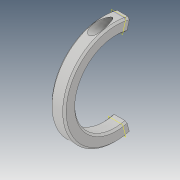
# Autodesk Inventor part: bottomCameraMount2
Saved by Autodesk Inventor 2018 (Build 220112000, 112)
## iProperties
Created: 2020-01-17
Part Number: bottomCameraMount2
Material: Generic
Document SubType Name: Modeling
Designer: anirudh
Density: 1 g/cm^3
Appearance: Default
Author: anirudh
Autodesk Inventor part; units mm, degrees
ref_plane "YZ Plane" through (0, 0, 0) normal (1, 0, 0) x (0, 1, 0)
ref_plane "XZ Plane" through (0, 0, 0) normal (0, 1, 0) x (-1, 0, 0)
ref_plane "XY Plane" through (0, 0, 0) normal (0, 0, 1) x (1, 0, 0)
sketch "Sketch1" plane through (0, 0, 0) normal (1, 0, 0) x (0, 1, 0)
  arc A0 (27.6013, -7.3958) -> (-27.6013, -7.3958) centre (0, 0) ccw
  arc A1 (35.894, -9.6178) -> (-35.894, -9.6178) centre (0, 0) ccw
  line L0 (27.6013, -7.3958) -> (35.894, -9.6178)
  line L1 (0, 0) -> (42.3648, 0) construction
  line L2 (-27.6013, -7.3958) -> (-35.894, -9.6178)
  line L3 (0, 0) -> (46.1302, 0) construction
  constraints: 8 end point, 4 point on circle, 2 centre point, 2 coincident, 2 horizontal
extrude "Extrusion1" add sketch "Sketch1" along normal blind 9.398
sketch "Sketch2" plane through (9.398, 35.894, -9.6178) normal (0, -0.258819, -0.9659258) x (-1, 0, 0)
  line L0 (0, -8.5852) -> (0, 0) projected
  line L1 (9.398, 0) -> (9.398, -8.5852) projected
  circle A0 centre (4.699, -4.2926) radius 1.8
  point P0 (9.398, -37.1602)
  dimension "d6" = 3.6
  constraints: 1 centre point
  measures "d6" diameter of A0
extrude "Extrusion2" cut sketch "Sketch2" against normal blind 25.4
ref_plane "Work Plane1" through (9.398, 36.6697, -6.7227) normal (0, -0.258819, -0.9659258) x (-1, 0, 0)
sketch "Sketch3" plane through (9.398, 36.6697, -6.7227) normal (0, -0.258819, -0.9659258) x (-1, 0, 0)
  circle A0 centre (4.699, -4.2926) radius 1.8 projected
  circle A1 centre (4.699, -4.2926) radius 3.556
  point P0 (9.398, -37.1602)
  dimension "d10" = 7.112
  constraints: 1 centre point, 1 coincident
  measures "d10" diameter of A1
extrude "Extrusion3" cut sketch "Sketch3" against normal blind 25.4 contours A0 | A1
sketch "Sketch4" plane through (9.398, -27.6013, -7.3958) normal (0, 0.258819, -0.9659258) x (-1, 0, 0)
  line L0 (9.398, 0) -> (0, 0) projected
  line L1 (9.398, -8.5852) -> (0, -8.5852) projected
  circle A0 centre (4.699, -4.2926) radius 1.8
  point P0 (9.398, 28.575)
  dimension "d13" = 3.6
  constraints: 1 centre point
  measures "d13" diameter of A0
extrude "Extrusion4" cut sketch "Sketch4" against normal blind 25.4
ref_plane "Work Plane2" through (9.398, -28.3771, -4.5007) normal (0, 0.258819, -0.9659258) x (-1, 0, 0)
sketch "Sketch5" plane through (9.398, -28.3771, -4.5007) normal (0, 0.258819, -0.9659258) x (-1, 0, 0)
  circle A0 centre (4.699, -4.2926) radius 1.8 projected
  circle A1 centre (4.699, -4.2926) radius 3.556
  point P0 (9.398, 28.575)
  dimension "d17" = 7.112
  constraints: 1 centre point, 1 coincident
  measures "d17" diameter of A1
extrude "Extrusion5" cut sketch "Sketch5" against normal blind 25.4 contours A0 | A1
sketch "Sketch6" plane through (9.398, 0, 0) normal (1, 0, 0) x (0, 0, -1)
  line L0 (7.3958, 27.6013) -> (9.6178, 35.894) projected
  arc A0 (7.3958, 27.6013) -> (7.3958, -27.6013) centre (0, 0) ccw
  arc A1 (9.6178, 35.894) -> (9.6178, -35.894) centre (0, 0) ccw
  line L1 (7.3958, 27.6013) -> (9.6178, 35.894)
  line L2 (9.6178, -35.894) -> (7.3958, -27.6013) projected
  line L3 (7.3958, -27.6013) -> (9.6178, -35.894)
  constraints: 4 end point, 4 point on circle, 2 centre point, 2 coincident, 2 collinear
extrude "Extrusion6" add sketch "Sketch6" along normal blind 0.381
sketch "Sketch7" plane through (0, 0, 0) normal (-1, 0, 0) x (0, 0, 1)
  arc A0 (-7.3958, -27.6013) -> (-7.3958, 27.6013) centre (0, 0) ccw projected
  arc A1 (-7.3958, -27.6013) -> (-7.3958, 27.6013) centre (0, 0) ccw
  arc A2 (-9.6178, -35.894) -> (-9.6178, 35.894) centre (0, 0) ccw projected
  arc A3 (-9.6178, -35.894) -> (-9.6178, 35.894) centre (0, 0) ccw
  line L0 (-9.6178, 35.894) -> (-7.3958, 27.6013) projected
  line L1 (-7.3958, 27.6013) -> (-9.6178, 35.894)
  line L2 (-7.3958, -27.6013) -> (-9.6178, -35.894) projected
  line L3 (-7.3958, -27.6013) -> (-9.6178, -35.894)
  constraints: 4 end point, 4 point on circle, 2 centre point, 2 coincident, 2 collinear
extrude "Extrusion7" add sketch "Sketch7" along normal blind 0.381
chamfer "Chamfer2" distance 1.27 angle 45 4 edges at (-0.381, 0, 37.1602) (9.779, 0, 37.1602) (9.779, 0, 28.575) (-0.381, 0, 28.575)
body "Solid1"
